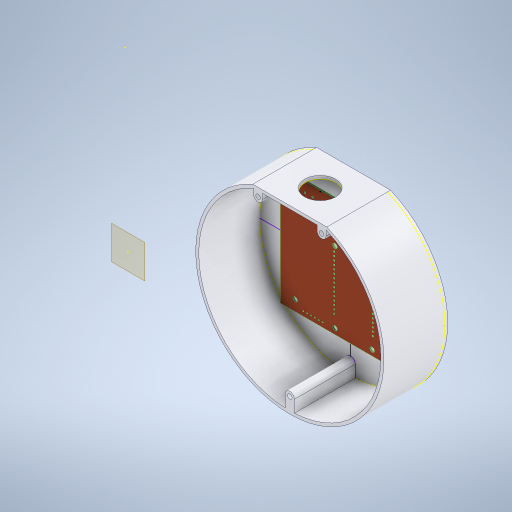
# Autodesk Inventor part: Modulo_DEC.kicad_pcb1
Saved by Autodesk Inventor 2023 (Build 270158000, 158)
## iProperties
Created: 2023-12-30
Part Number: Modulo_DEC.kicad_pcb1
Material: Generic
Document SubType Name: Modeling
Designer: Usuario
Density: 1 g/cm^3
Appearance: Board Outline
Author: Usuario
Autodesk Inventor part; units mm, degrees
ref_plane "YZ Plane" through (0, 0, 0) normal (1, 0, 0) x (0, 1, 0)
ref_plane "XZ Plane" through (0, 0, 0) normal (0, 1, 0) x (-1, 0, 0)
ref_plane "XY Plane" through (0, 0, 0) normal (0, 0, 1) x (1, 0, 0)
sketch "Sketch1" plane through (0, 0, 0) normal (0, 0, 1) x (1, 0, 0)
  line L0 (190.01, 101.6) -> (103.121, 101.6)
  line L1 (103.121, 101.6) -> (103.121, 24)
  line L2 (103.121, 24) -> (190.01, 24)
  circle A0 centre (180.571, 84.064) radius 1.5
  circle A1 centre (113.096, 84.014) radius 1.5
  circle A2 centre (113.096, 31.014) radius 1.5
  circle A3 centre (168.406, 95.094) radius 0.66
  circle A4 centre (173.406, 95.094) radius 0.66
  circle A5 centre (178.406, 95.094) radius 0.66
  circle A6 centre (183.406, 95.094) radius 0.66
  circle A7 centre (152.121, 95.089) radius 0.66
  circle A8 centre (157.121, 95.089) radius 0.66
  circle A9 centre (162.121, 95.089) radius 0.66
  circle A10 centre (135.871, 95.089) radius 0.66
  circle A11 centre (140.871, 95.089) radius 0.66
  circle A12 centre (145.871, 95.089) radius 0.66
  circle A13 centre (119.586, 95.094) radius 0.66
  circle A14 centre (124.586, 95.094) radius 0.66
  circle A15 centre (129.586, 95.094) radius 0.66
  circle A16 centre (108.096, 95.014) radius 0.66
  circle A17 centre (113.096, 95.014) radius 0.66
  circle A18 centre (140.746, 84.684) radius 0.7
  circle A19 centre (145.826, 84.684) radius 0.7
  circle A20 centre (118.436, 27.064) radius 0.4
  circle A21 centre (120.976, 27.064) radius 0.4
  circle A22 centre (123.516, 27.064) radius 0.4
  circle A23 centre (126.056, 27.064) radius 0.4
  circle A24 centre (128.596, 27.064) radius 0.4
  circle A25 centre (131.136, 27.064) radius 0.4
  circle A26 centre (185.311, 77.939) radius 0.4
  circle A27 centre (182.771, 77.939) radius 0.4
  circle A28 centre (180.231, 77.939) radius 0.4
  circle A29 centre (177.691, 77.939) radius 0.4
  circle A30 centre (175.151, 77.939) radius 0.4
  circle A31 centre (172.611, 77.939) radius 0.4
  circle A32 centre (164.23, 35.66) radius 0.51
  circle A33 centre (164.23, 38.2) radius 0.51
  circle A34 centre (164.23, 40.74) radius 0.51
  circle A35 centre (164.23, 43.28) radius 0.51
  circle A36 centre (164.23, 45.82) radius 0.51
  circle A37 centre (164.23, 48.36) radius 0.51
  circle A38 centre (164.23, 50.9) radius 0.51
  circle A39 centre (164.23, 53.44) radius 0.51
  circle A40 centre (164.23, 55.98) radius 0.51
  circle A41 centre (164.23, 58.52) radius 0.51
  circle A42 centre (164.23, 61.06) radius 0.51
  circle A43 centre (164.23, 63.6) radius 0.51
  circle A44 centre (164.23, 66.14) radius 0.51
  circle A45 centre (164.23, 68.68) radius 0.51
  circle A46 centre (164.23, 71.22) radius 0.51
  circle A47 centre (138.83, 71.22) radius 0.51
  circle A48 centre (138.83, 68.68) radius 0.51
  circle A49 centre (138.83, 66.14) radius 0.51
  circle A50 centre (138.83, 63.6) radius 0.51
  circle A51 centre (138.83, 61.06) radius 0.51
  circle A52 centre (138.83, 58.52) radius 0.51
  circle A53 centre (138.83, 55.98) radius 0.51
  circle A54 centre (138.83, 53.44) radius 0.51
  circle A55 centre (138.83, 50.9) radius 0.51
  circle A56 centre (138.83, 48.36) radius 0.51
  circle A57 centre (138.83, 45.82) radius 0.51
  circle A58 centre (138.83, 43.28) radius 0.51
  circle A59 centre (138.83, 40.74) radius 0.51
  circle A60 centre (138.83, 38.2) radius 0.51
  circle A61 centre (138.83, 35.66) radius 0.51
  circle A62 centre (163.81, 27.7) radius 1.5
  circle A63 centre (163.81, 74.65) radius 1.5
  circle A64 centre (139.3, 27.7) radius 1.5
  circle A65 centre (139.3, 74.65) radius 1.5
  line L3 (190.01, 24) -> (190.01, 101.6)
  point P0 (146.5655, 62.8)
  constraints: 66 centre point, 8 end point
extrude "Extrusion2" add sketch "Sketch1" along normal blind 1
ref_plane "Work Plane1" through (0, 0, -2) normal (0, 0, 1) x (1, 0, 0)
sketch "Sketch3" plane through (0, 0, -2) normal (0, 0, 1) x (1, 0, 0)
  line L0 (190.01, 101.6) -> (103.121, 101.6) projected
  line L1 (103.121, 24) -> (190.01, 24) projected
  line L2 (190.01, 24) -> (190.01, 101.6) projected
  line L3 (103.121, 101.6) -> (103.121, 24) projected
  circle A0 centre (146.5655, 62.8) radius 60
  line L4 (146.5655, 122.8) -> (146.5655, 119.8)
  line L5 (146.5655, 119.8) -> (165.3005, 119.8)
  line L6 (146.5655, 119.8) -> (127.8305, 119.8)
  line L7 (165.3005, 119.8) -> (168.2911, 119.8)
  line L8 (127.8305, 119.8) -> (124.8399, 119.8)
  line L9 (146.5655, 119.8) -> (146.5655, 117.8)
  line L10 (146.5655, 117.8) -> (172.9473, 117.8)
  line L11 (146.5655, 117.8) -> (120.1837, 117.8)
  circle A1 centre (146.5655, 62.8) radius 62
  line L12 (124.8399, 119.8) -> (122.1729, 119.8)
  line L13 (120.1837, 117.8) -> (117.9473, 117.8)
  line L14 (168.2911, 119.8) -> (170.9581, 119.8)
  line L15 (172.9473, 117.8) -> (175.1837, 117.8)
  point P0 (0, 0)
  point P1 (122.5863, 117.8)
  point P2 (170.5447, 117.8)
  dimension "d15" = 3
  dimension "d16" = 2
  constraints: 24 end point, 8 point on line, 7 point on circle, 2 centre point, 2 perpendicular, 1 coincident, 1 parallel, 1 vertical
  measures "d15" distance of L4.start L4.end
  measures "d16" distance of L4.end L9.end
extrude "Extrusion3" add sketch "Sketch3" against normal blind 2 separate body contours L2 L1 L3 L0 | A0 L11 L10
extrude "Extrusion6" add sketch "Sketch3" against normal blind 2 contours L7 L14 A1 L15 L10 A0 | A0 L10 L9 L5 | L10 L15 A1 L13 L11 A0 | L9 L11 A0 L6 | A0 L11 L13 A1 L12 L8 bodies 2
extrude "Extrusion7" add sketch "Sketch3" along normal blind 40 contours L7 L14 A1 L15 L10 A0 | A0 L10 L9 L5 | L10 L15 A1 L13 L11 A0 | L9 L11 A0 L6 | A0 L11 L13 A1 L12 L8 bodies 2
sketch "Sketch4" plane through (122.5863, 117.8, -2) normal (0, -1, 0) x (1, 0, 0)
  circle A0 centre (23.9792, 20) radius 10.2
  line L0 (30.7802, 31.7) -> (37.5122, 19.9601)
  line L1 (37.5122, 19.9601) -> (30.7111, 8.2601)
  line L2 (30.7111, 8.2601) -> (17.1781, 8.3)
  line L3 (17.1781, 8.3) -> (10.4461, 20.0399)
  line L4 (10.4461, 20.0399) -> (17.2472, 31.7399)
  line L5 (17.2472, 31.7399) -> (30.7802, 31.7)
  point P0 (-122.5863, 2)
  constraints: 12 end point, 1 centre point, 1 coincident, 13 other
extrude "Extrusion8" cut sketch "Sketch4" against normal blind 60 contours A0 bodies 2
sketch "Sketch5" plane through (0, 0, -2) normal (0, 0, 1) x (1, 0, 0)
  circle A0 centre (113.096, 84.014) radius 1.5 projected
  circle A1 centre (113.096, 84.014) radius 1.5
  circle A2 centre (180.571, 84.064) radius 1.5 projected
  circle A3 centre (180.571, 84.064) radius 1.5
  circle A4 centre (113.096, 31.014) radius 1.5 projected
  circle A5 centre (113.096, 31.014) radius 1.5
  point P0 (0, 0)
  constraints: 3 centre point, 3 coincident
extrude "Extrusion9" cut sketch "Sketch5" against normal blind 60 bodies 2
sketch "Sketch7" plane through (0, 0, -2) normal (0, 0, 1) x (1, 0, 0)
  circle A0 centre (146.57, 10.8434) radius 3.0673
  line L0 (143.5028, 10.8093) -> (143.5028, 2.8782)
  arc A1 (122.5863, 117.8) -> (170.5447, 117.8) centre (146.5655, 62.8) ccw projected
  line L1 (149.6373, 10.8434) -> (149.6373, 2.8787)
  arc A2 (122.1729, 119.8) -> (170.9581, 119.8) centre (146.5655, 62.8) ccw projected
  line L2 (84.5655, 62.7864) -> (208.5655, 62.7864)
  line L3 (122.5863, 117.8) -> (170.5447, 117.8) projected
  circle A3 centre (125.641, 114.4161) radius 3
  line L4 (122.641, 114.4161) -> (122.641, 117.8)
  line L5 (128.641, 114.4161) -> (128.641, 117.8)
  line L6 (170.5447, 117.8) -> (122.5863, 117.8) projected
  line L7 (146.5655, 2.8) -> (146.5655, 117.8)
  circle A4 centre (167.49, 114.4161) radius 3
  line L8 (170.49, 114.4161) -> (170.49, 117.8)
  line L9 (164.49, 114.4161) -> (164.49, 117.8)
  circle A5 centre (125.641, 114.4161) radius 1.5
  circle A6 centre (167.49, 114.4161) radius 1.5
  point P0 (0, 0)
  constraints: 16 end point, 11 point on circle, 5 centre point, 5 symmetric about line, 2 coincident, 2 point on line, 2 tangent, 2 vertical, 1 horizontal, 1 midpoint, 1 parallel, 1 perpendicular, 1 other
extrude "Extrusion10" add sketch "Sketch7" along normal blind 40 contours A0 L7 | L1 A1 L7 A0 | L7 A0 | L7 A1 L0 A0 bodies 2
sketch "Sketch8" plane through (0, 0, 38) normal (0, 0, 1) x (1, 0, 0)
  arc A0 (149.6373, 10.8434) -> (143.5028, 10.8093) centre (146.57, 10.8434) ccw projected
  circle A1 centre (146.57, 10.8434) radius 1.5
  point P0 (0, 0)
  dimension "d32" = 3
  constraints: 1 centre point, 1 coincident
  measures "d32" diameter of A1
extrude "Extrusion11" cut sketch "Sketch8" against normal blind 5 bodies 2
extrude "Extrusion12" add sketch "Sketch7" along normal blind 40 contours L5 A3 L4 L3 | L3 L8 A4 L9 | A3 | A4 bodies 2
sketch "Sketch9" plane through (128.641, 117.8, 38) normal (0, -1, 0) x (1, 0, 0)
  circle A0 centre (17.9245, -20) radius 10.2 projected
  line L0 (24.6743, -8.309) -> (31.4241, -20)
  line L1 (31.4241, -20) -> (24.6743, -31.691)
  line L2 (24.6743, -31.691) -> (11.1747, -31.691)
  line L3 (11.1747, -31.691) -> (4.4249, -20)
  line L4 (4.4249, -20) -> (11.1747, -8.309)
  line L5 (11.1747, -8.309) -> (24.6743, -8.309)
  point P0 (-128.641, -38)
  constraints: 12 end point, 1 coincident, 13 other
extrude "Extrusion13" add sketch "Sketch7" along normal blind 35 contours A5 | A6 bodies 2
ref_plane "Work Plane6" through (84.5655, 62.8, -2) normal (-1, 0, 0) x (0, 0, 1)
sketch "Sketch10" plane through (84.5655, 62.8, -2) normal (-1, 0, 0) x (0, 0, 1)
  circle A0 centre (20, 35) radius 1.5
  point P0 (2, -62.8)
  dimension "d43" = 3
  constraints: 1 centre point
  measures "d43" diameter of A0
extrude "Extrusion14" cut sketch "Sketch10" against normal blind 35 bodies 2
body "Solid1"
body "Solid2"
